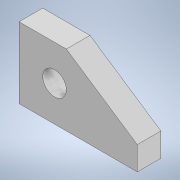
# Autodesk Inventor part: Exercício1.2
Saved by Autodesk Inventor 2022 (Build 260153000, 153)
## iProperties
Created: 2023-03-07
Part Number: Exercício1.2
Material: Genérico
Document SubType Name: Modeling
Designer: jpjoa
Density: 1 g/cm^3
Appearance: Padrão
Author: jpjoa
Autodesk Inventor part; units mm, degrees
ref_plane "YZ Plane" through (0, 0, 0) normal (1, 0, 0) x (0, 1, 0)
ref_plane "XZ Plane" through (0, 0, 0) normal (0, 1, 0) x (-1, 0, 0)
ref_plane "XY Plane" through (0, 0, 0) normal (0, 0, 1) x (1, 0, 0)
sketch "Esboço1" plane through (0, 0, 0) normal (0, 0, 1) x (1, 0, 0)
  line L0 (0, 0) -> (50, 0)
  line L1 (0, 0) -> (0, 30)
  line L2 (0, 30) -> (20, 30)
  line L3 (50, 0) -> (50, 10)
  line L4 (50, 10) -> (20, 30)
  circle A0 centre (15, 15) radius 5
  dimension "d0" = 50
  dimension "d1" = 30
  dimension "d2" = 20
  dimension "d3" = 10
  dimension "d4" = 10
  dimension "d5" = 15
  dimension "d6" = 15
  constraints: 10 end point, 2 vertical, 1 centre point, 1 horizontal, 1 perpendicular
  measures "d0" distance of L0.start L0.end
  measures "d1" distance of L0.start L1.end
  measures "d2" distance of L1.end L2.end
  measures "d3" distance of L0.end L3.end
  measures "d4" diameter of A0
  measures "d5" distance from line of A0.centre L0
  measures "d6" distance from line of A0.centre L1
extrude "Extrusão1" add sketch "Esboço1" along normal blind 10
